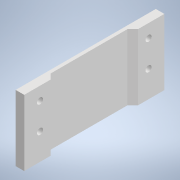
# Autodesk Inventor part: wheelguard
Saved by Autodesk Inventor 2020.1 (Build 241239000, 239)
## iProperties
Created: 2019-12-06
Part Number: wheelguard
Material: Generic
Document SubType Name: Modeling
Designer: tbloo
Density: 1 g/cm^3
Appearance: Default
Author: tbloo
Autodesk Inventor part; units mm, degrees
ref_plane "YZ Plane" through (0, 0, 0) normal (1, 0, 0) x (0, 1, 0)
ref_plane "XZ Plane" through (0, 0, 0) normal (0, 1, 0) x (-1, 0, 0)
ref_plane "XY Plane" through (0, 0, 0) normal (0, 0, 1) x (1, 0, 0)
sketch "Sketch1" plane through (0, 0, 0) normal (1, 0, 0) x (0, 1, 0)
  line L0 (24, 0) -> (64, 0)
  line L1 (64, 0) -> (64, 85)
  line L2 (64, 85) -> (24, 85)
  line L3 (24, -2) -> (24, 0)
  line L4 (24, 0) -> (24, 85)
  line L5 (24, 0) -> (109, 0) construction
  point P0 (0, 0)
  dimension "d1" = 85
  dimension "d13" = 90
  constraints: 12 end point, 2 horizontal, 2 perpendicular, 1 parallel, 1 vertical, 2 other
  measures "d1" distance of L1.end L0.end
  measures "d13" angle of L5 L4
extrude "Extrusion1" add sketch "Sketch1" along normal blind 2
sketch "Sketch2" plane through (2, 0, 0) normal (1, 0, 0) x (0, 0, -1)
  circle A0 centre (-75.4, 56) radius 1.85
  circle A1 centre (-75.4, 40) radius 1.85
  circle A2 centre (-9.6, 56) radius 1.85
  circle A3 centre (-9.6, 40) radius 1.85
  line L0 (-69, 24) -> (-69, 64)
  line L1 (-16, 24) -> (-16, 64)
  line L2 (-16, 0) -> (48, 0) construction
  line L3 (-85, 64) -> (-85, 24)
  line L4 (-69, 64) -> (-85, 64)
  line L5 (-85, 64) -> (-85, 24)
  line L6 (-69, 24) -> (-69, 64)
  line L7 (0, 24) -> (0, 64)
  line L8 (-16, 64) -> (0, 64)
  line L9 (0, 64) -> (0, 24)
  line L10 (-16, 24) -> (-16, 64)
  line L11 (-85, 24) -> (0, 24)
  point P0 (-69, 0)
  dimension "d5" = 90
  constraints: 24 end point, 4 centre point, 2 point on line, 1 horizontal
  measures "d5" angle of L2 L1
extrude "Extrusion2" add sketch "Sketch2" along normal blind 3.2
chamfer "Chamfer1" distance 3.175 angle 45 2 edges at (2, 44, 16) (2, 44, 69)
sketch "Sketch3" plane through (5.2, 0, 0) normal (1, 0, 0) x (0, 0, -1)
  circle A0 centre (-75.4, 56) radius 1.85
  circle A1 centre (-75.4, 40) radius 1.85
  circle A2 centre (-9.6, 40) radius 1.85
  circle A3 centre (-9.6, 56) radius 1.85
  point P0 (0, 0)
  constraints: 4 centre point
extrude "Extrusion3" cut sketch "Sketch3" against normal through all
body "Solid1"
